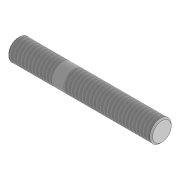
# Autodesk Inventor part: Bottom
Saved by Autodesk Inventor 2022.5 (Build 265521000, 521)
## iProperties
Created: 2020-02-29
Part Number: Bottom
Document SubType Name: Modeling
Designer: Administrator
Density: 1 g/cm^3
Material: Generic
Appearance: Default
Author: Administrator
Autodesk Inventor part; units mm, degrees
ref_plane "YZ Plane" through (0, 0, 0) normal (1, 0, 0) x (0, 1, 0)
ref_plane "XZ Plane" through (0, 0, 0) normal (0, 1, 0) x (-1, 0, 0)
ref_plane "XY Plane" through (0, 0, 0) normal (0, 0, 1) x (1, 0, 0)
sketch "Sketch2" plane through (0, 0, 0) normal (1, 0, 0) x (0, 1, 0)
  circle A0 centre (0, 0) radius 1.5
  dimension "d9" = 3
  constraints: 1 centre point, 1 coincident
  measures "d9" diameter of A0
extrude "Extrusion2" add sketch "Sketch2" along normal blind 20
chamfer "Chamfer1" distance 0.2 angle 45 2 edges at (0, -1.5, 0) (20, -1.5, 0)
thread "Thread1" size "M3x0.5" class "6g" standard "ANSI Metric M Profile" length 6
thread "Thread2" size "M3x0.5" class "6g" standard "ANSI Metric M Profile" length 12
body "Solid2"
